ScrewMount_v5 (Autodesk Fusion 360 design; units mm, degrees)
Autodesk Fusion 360 part; units mm, degrees
sketch "Sketch1" plane through (0, 0, 0) normal (0, 0, 1) x (1, 0, 0)
  line L0 (0, 0) -> (0, 8)
  line L1 (0, 0) -> (8, 0)
  line L2 (8, 0) -> (8, 8)
  line L3 (8, 8) -> (0, 8)
  dimension "d1" = 8
  dimension "d2" = 8
  constraint coincident L0.start L1.start
  constraint vertical L0
  constraint perpendicular L0 L1
  constraint perpendicular L1 L2
  measures "d1" distance of L0.start L0.end
  measures "d2" distance of L0.start L1.end
extrude "Extrude1" add sketch "Sketch1" along normal blind 2.4
sketch "Sketch2" plane through (0, 0, 2.4) normal (0, 0, 1) x (-1, 0, 0)
  line L0 (0, 0) -> (-8, 0)
  line L1 (-8, 0) -> (-8, -8)
  line L2 (-8, -8) -> (0, -8)
  line L3 (0, -8) -> (0, 0)
  line L4 (-8, -8) -> (0, 0)
  line L5 (-8, 0) -> (0, -8)
  line L6 (-6.8, -5.6166) -> (-4, -7.2332)
  line L7 (-4, -7.2332) -> (-1.2, -5.6166)
  line L8 (-1.2, -5.6166) -> (-1.2, -2.3834)
  line L9 (-1.2, -2.3834) -> (-4, -0.7668)
  line L10 (-4, -0.7668) -> (-6.8, -2.3834)
  line L11 (-6.8, -2.3834) -> (-6.8, -5.6166)
  point P0 (-4, -4)
  dimension "d5" = 2.8
  constraint coincident L1.end L2.start
  constraint coincident L0.start L3.end
  constraint coincident L0.end L1.start
  constraint coincident L2.end L3.start
  constraint midpoint L4 P0
  measures "d5" distance of P0 L11
extrude "Extrude2" add sketch "Sketch2" along normal blind 2 contours L0 L4 L5 L9 L10 | L3 L4 L5 L7 L8 L9 | L1 L4 L5 L6 L10 L11 | L2 L4 L5 L6 L7
sketch "Sketch3" plane through (0, 0, 2.4) normal (0, 0, 1) x (-1, 0, 0)
  line L0 (-6.8, -5.6166) -> (-4, -7.2332)
  line L1 (-4, -7.2332) -> (-1.2, -5.6166)
  line L2 (-1.2, -5.6166) -> (-1.2, -2.3834)
  line L3 (-1.2, -2.3834) -> (-4, -0.7668)
  line L4 (-4, -0.7668) -> (-6.8, -2.3834)
  line L5 (-6.8, -2.3834) -> (-6.8, -5.6166)
  circle A0 centre (-4, -4) radius 1.7
  dimension "d12" = 3.4
  measures "d12" diameter of A0
extrude "Extrude3" cut sketch "Sketch3" against normal blind 2.4 contours A0
sketch "Sketch4" plane through (0, 0, 0) normal (0, -1, 0) x (1, 0, 0)
  line L0 (0, 0) -> (8, 0)
  line L1 (8, 0) -> (8, 4.4)
  line L2 (8, 4.4) -> (0, 4.4)
  line L3 (0, 4.4) -> (0, 0)
  line L4 (8, 4.4) -> (0, 4.4)
  line L5 (0, 4.4) -> (0, 0)
  line L6 (0, 0) -> (8, 0)
  line L7 (8, 0) -> (8, 4.4)
  constraint horizontal L4
  constraint vertical L5
  constraint horizontal L6
  constraint vertical L7
  constraint coincident L0.start L3.end
  constraint coincident L1.end L2.start
extrude "Extrude4" add sketch "Sketch4" along normal blind 1
sketch "Sketch5" plane through (0, 0, 0) normal (-1, 0, 0) x (0, -1, 0)
  line L0 (-8, 0) -> (1, 0)
  line L1 (1, 0) -> (1, 4.4)
  line L2 (1, 4.4) -> (-8, 4.4)
  line L3 (-8, 4.4) -> (-8, 0)
